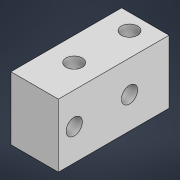
# Autodesk Inventor part: 200522
Saved by Autodesk Inventor 2022.2 (Build 262287000, 287)
## iProperties
Created: 2022-09-19
Part Number: 200522
Material: Generic
Document SubType Name: Modeling
Designer: robotics
Mass: 18.5328 g
Surface Area: 64.7474 cm^2
Volume: 18.5328 cm^3
Density: 1 g/cm^3
Appearance: Default
Author: robotics
Autodesk Inventor part; units mm, degrees
ref_plane "YZ Plane" through (0, 0, 0) normal (1, 0, 0) x (0, 1, 0)
ref_plane "XZ Plane" through (0, 0, 0) normal (0, 1, 0) x (-1, 0, 0)
ref_plane "XY Plane" through (0, 0, 0) normal (0, 0, 1) x (1, 0, 0)
sketch "Sketch1" plane through (0, 0, 0) normal (0, 1, 0) x (-1, 0, 0)
  line L0 (0, 0) -> (19.05, 0)
  line L1 (19.05, 0) -> (19.05, 44.45)
  line L2 (19.05, 44.45) -> (0, 44.45)
  line L3 (0, 44.45) -> (0, 0)
  dimension "d0" = 19.05
  dimension "d1" = 44.45
  constraints: 8 end point, 2 parallel, 1 horizontal, 1 perpendicular
  measures "d0" distance of L1.end L2.end
  measures "d1" distance of L0.end L1.end
extrude "Extrusion1" add sketch "Sketch1" along normal blind 25.4
sketch "Sketch2" plane through (0, 0, 44.45) normal (1, 0, 0) x (0, 0, -1)
  line L0 (0, 0) -> (44.45, 0) projected
  line L1 (0, 0) -> (0, 25.4) projected
  line L2 (44.45, 0) -> (44.45, 25.4) projected
  point P0 (6.35, 12.7)
  point P1 (34.925, 12.7)
  point P2 (44.45, 12.7)
  dimension "d4" = 12.7
  dimension "d5" = 12.7
  dimension "d6" = 6.35
  dimension "d7" = 9.525
  constraints: 1 midpoint
  measures "d4" distance from line of L0 point (6.35, 12.7)
  measures "d5" distance from line of L0 point (34.925, 12.7)
  measures "d6" distance from line of L1 point (6.35, 12.7)
  measures "d7" distance of point (44.45, 12.7) point (34.925, 12.7)
hole "Hole1" at (0, 12.7, 38.1) direction (-1, 0, 0) diameter 6.5278 depth 50.8 tip angle 118
sketch "Sketch3" plane through (0, 0, 0) normal (0, -1, 0) x (1, 0, 0)
  line L0 (0, 44.45) -> (0, 0) projected
  line L1 (-19.05, 44.45) -> (0, 44.45) projected
  point P0 (-9.525, 28.575)
  point P1 (-9.525, 9.6957)
  dimension "d15" = 9.525
  dimension "d16" = 15.875
  measures "d15" distance from line of L0 point (-9.525, 28.575)
  measures "d16" distance from line of L1 point (-9.525, 28.575)
hole "Hole2" at (-9.525, 0, 28.575) direction (0, 1, 0) diameter 6.5278 depth 50.8 tip angle 118
sketch "Sketch4" plane through (0, 0, 44.45) normal (1, 0, 0) x (0, 0, -1)
  line L0 (0, 25.4) -> (44.45, 25.4) projected
  line L1 (0, 0) -> (0, 25.4) projected
  point P0 (44.45, 0)
  point P1 (28.575, 12.7)
  dimension "d24" = 12.7
  dimension "d25" = 28.575
  measures "d24" distance from line of L0 point (28.575, 12.7)
  measures "d25" distance from line of point (28.575, 12.7) L1
sketch "Sketch5" plane through (0, 0, 0) normal (0, -1, 0) x (1, 0, 0)
  line L0 (0, 44.45) -> (0, 0) projected
  line L1 (0, 0) -> (-19.05, 0) projected
  point P0 (-9.525, 6.35)
  dimension "d26" = 9.525
  dimension "d27" = 6.35
  measures "d26" distance from line of L0 point (-9.525, 6.35)
  measures "d27" distance from line of L1 point (-9.525, 6.35)
hole "Hole3" at (-9.525, 0, 6.35) direction (0, 1, 0) diameter 6.5278 depth 50.8 tip angle 118
hole "Hole4" at (0, 12.7, 15.875) direction (-1, 0, 0) diameter 6.5278 depth 50.8 tip angle 118
body "Solid1"
